Autodesk Fusion 360 part; units mm, degrees
(part 37 of 40)
  line L10333 (174.0805, 208.06) -> (173.9342, 208.1383) construction
  line L10334 (173.9342, 208.1383) -> (173.7873, 208.216) construction
  line L10335 (173.7873, 208.216) -> (173.6399, 208.2931) construction
  line L10336 (173.6399, 208.2931) -> (173.4919, 208.3695) construction
  line L10337 (173.4919, 208.3695) -> (173.3434, 208.4453) construction
  line L10338 (173.3434, 208.4453) -> (173.1943, 208.5205) construction
  line L10339 (173.1943, 208.5205) -> (173.0447, 208.595) construction
  line L10340 (173.0447, 208.595) -> (172.8946, 208.669) construction
  line L10341 (172.8946, 208.669) -> (172.7439, 208.7423) construction
  line L10342 (172.7439, 208.7423) -> (172.5927, 208.8149) construction
  line L10343 (172.5927, 208.8149) -> (172.4411, 208.887) construction
  line L10344 (172.4411, 208.887) -> (172.2889, 208.9584) construction
  line L10345 (172.2889, 208.9584) -> (172.1667, 209.0151) construction
  line L10346 (172.1667, 209.0151) -> (172.0748, 209.0573) construction
  line L10347 (172.0748, 209.0573) -> (172.0135, 209.0853) construction
  line L10348 (172.0135, 209.0853) -> (171.9828, 209.0993) construction
  spline S138 degree 5 poles (217.8271, 89.2315) (217.8299, 89.2007) (217.8349, 89.1391) (217.8398, 89.0467) (217.8417, 88.9234) (217.8376, 88.769) (217.8289, 88.6144) (217.8174, 88.4597) (217.8043, 88.305) (217.7903, 88.1502) (217.7751, 87.9955) (217.7585, 87.8407) (217.74, 87.686) (217.7191, 87.5312) (217.6961, 87.3765) (217.671, 87.2218) (217.6441, 87.0671) (217.6158, 86.9125) (217.5862, 86.7579) (217.5553, 86.6034) (217.5233, 86.4489) (217.4899, 86.2945) (217.4552, 86.1402) (217.4191, 85.986) (217.3817, 85.8318) (217.3429, 85.6778) (217.3029, 85.5238) (217.2617, 85.3699) (217.2193, 85.2161) (217.1759, 85.0624) (217.1313, 84.9088) (217.0856, 84.7553) (217.0388, 84.602) (216.9909, 84.4487) (216.9419, 84.2956) (216.8919, 84.1426) (216.8407, 83.9897) (216.7886, 83.8369) (216.7355, 83.6842) (216.6813, 83.5317) (216.6262, 83.3794) (216.57, 83.2271) (216.513, 83.075) (216.4549, 82.923) (216.3959, 82.7712) (216.3359, 82.6196) (216.275, 82.468) (216.2132, 82.3167) (216.1505, 82.1655) (216.0868, 82.0144) (216.0223, 81.8635) (215.9569, 81.7128) (215.8905, 81.5622) (215.8233, 81.4118) (215.7553, 81.2616) (215.6863, 81.1115) (215.6166, 80.9616) (215.5459, 80.8119) (215.4745, 80.6624) (215.4021, 80.513) (215.329, 80.3638) (215.255, 80.2148) (215.1802, 80.066) (215.1046, 79.9174) (215.0282, 79.7689) (214.951, 79.6207) (214.873, 79.4726) (214.7942, 79.3248) (214.7146, 79.1771) (214.6343, 79.0297) (214.5531, 78.8824) (214.4876, 78.7648) (214.4381, 78.6766) (214.4049, 78.6179) (214.3883, 78.5885) knots 0 0 0 0 0 0 0.01428571 0.02857143 0.04285714 0.05714286 0.07142857 0.08571429 0.1 0.11428571 0.12857143 0.14285714 0.15714286 0.17142857 0.18571429 0.2 0.21428571 0.22857143 0.24285714 0.25714286 0.27142857 0.28571429 0.3 0.31428571 0.32857143 0.34285714 0.35714286 0.37142857 0.38571429 0.4 0.41428571 0.42857143 0.44285714 0.45714286 0.47142857 0.48571429 0.5 0.51428571 0.52857143 0.54285714 0.55714286 0.57142857 0.58571429 0.6 0.61428571 0.62857143 0.64285714 0.65714286 0.67142857 0.68571429 0.7 0.71428571 0.72857143 0.74285714 0.75714286 0.77142857 0.78571429 0.8 0.81428571 0.82857143 0.84285714 0.85714286 0.87142857 0.88571429 0.9 0.91428571 0.92857143 0.94285714 0.95714286 0.97142857 0.98571429 1 1 1 1 1 1
  line L10349 (217.8271, 89.2315) -> (217.8299, 89.2007) construction
  line L10350 (217.8299, 89.2007) -> (217.8349, 89.1391) construction
  line L10351 (217.8349, 89.1391) -> (217.8398, 89.0467) construction
  line L10352 (217.8398, 89.0467) -> (217.8417, 88.9234) construction
  line L10353 (217.8417, 88.9234) -> (217.8376, 88.769) construction
  line L10354 (217.8376, 88.769) -> (217.8289, 88.6144) construction
  line L10355 (217.8289, 88.6144) -> (217.8174, 88.4597) construction
  line L10356 (217.8174, 88.4597) -> (217.8043, 88.305) construction
  line L10357 (217.8043, 88.305) -> (217.7903, 88.1502) construction
  line L10358 (217.7903, 88.1502) -> (217.7751, 87.9955) construction
  line L10359 (217.7751, 87.9955) -> (217.7585, 87.8407) construction
  line L10360 (217.7585, 87.8407) -> (217.74, 87.686) construction
  line L10361 (217.74, 87.686) -> (217.7191, 87.5312) construction
  line L10362 (217.7191, 87.5312) -> (217.6961, 87.3765) construction
  line L10363 (217.6961, 87.3765) -> (217.671, 87.2218) construction
  line L10364 (217.671, 87.2218) -> (217.6441, 87.0671) construction
  line L10365 (217.6441, 87.0671) -> (217.6158, 86.9125) construction
  line L10366 (217.6158, 86.9125) -> (217.5862, 86.7579) construction
  line L10367 (217.5862, 86.7579) -> (217.5553, 86.6034) construction
  line L10368 (217.5553, 86.6034) -> (217.5233, 86.4489) construction
  line L10369 (217.5233, 86.4489) -> (217.4899, 86.2945) construction
  line L10370 (217.4899, 86.2945) -> (217.4552, 86.1402) construction
  line L10371 (217.4552, 86.1402) -> (217.4191, 85.986) construction
  line L10372 (217.4191, 85.986) -> (217.3817, 85.8318) construction
  line L10373 (217.3817, 85.8318) -> (217.3429, 85.6778) construction
  line L10374 (217.3429, 85.6778) -> (217.3029, 85.5238) construction
  line L10375 (217.3029, 85.5238) -> (217.2617, 85.3699) construction
  line L10376 (217.2617, 85.3699) -> (217.2193, 85.2161) construction
  line L10377 (217.2193, 85.2161) -> (217.1759, 85.0624) construction
  line L10378 (217.1759, 85.0624) -> (217.1313, 84.9088) construction
  line L10379 (217.1313, 84.9088) -> (217.0856, 84.7553) construction
  line L10380 (217.0856, 84.7553) -> (217.0388, 84.602) construction
  line L10381 (217.0388, 84.602) -> (216.9909, 84.4487) construction
  line L10382 (216.9909, 84.4487) -> (216.9419, 84.2956) construction
  line L10383 (216.9419, 84.2956) -> (216.8919, 84.1426) construction
  line L10384 (216.8919, 84.1426) -> (216.8407, 83.9897) construction
  line L10385 (216.8407, 83.9897) -> (216.7886, 83.8369) construction
  line L10386 (216.7886, 83.8369) -> (216.7355, 83.6842) construction
  line L10387 (216.7355, 83.6842) -> (216.6813, 83.5317) construction
  line L10388 (216.6813, 83.5317) -> (216.6262, 83.3794) construction
  line L10389 (216.6262, 83.3794) -> (216.57, 83.2271) construction
  line L10390 (216.57, 83.2271) -> (216.513, 83.075) construction
  line L10391 (216.513, 83.075) -> (216.4549, 82.923) construction
  line L10392 (216.4549, 82.923) -> (216.3959, 82.7712) construction
  line L10393 (216.3959, 82.7712) -> (216.3359, 82.6196) construction
  line L10394 (216.3359, 82.6196) -> (216.275, 82.468) construction
  line L10395 (216.275, 82.468) -> (216.2132, 82.3167) construction
  line L10396 (216.2132, 82.3167) -> (216.1505, 82.1655) construction
  line L10397 (216.1505, 82.1655) -> (216.0868, 82.0144) construction
  line L10398 (216.0868, 82.0144) -> (216.0223, 81.8635) construction
  line L10399 (216.0223, 81.8635) -> (215.9569, 81.7128) construction
  line L10400 (215.9569, 81.7128) -> (215.8905, 81.5622) construction
  line L10401 (215.8905, 81.5622) -> (215.8233, 81.4118) construction
  line L10402 (215.8233, 81.4118) -> (215.7553, 81.2616) construction
  line L10403 (215.7553, 81.2616) -> (215.6863, 81.1115) construction
  line L10404 (215.6863, 81.1115) -> (215.6166, 80.9616) construction
  line L10405 (215.6166, 80.9616) -> (215.5459, 80.8119) construction
  line L10406 (215.5459, 80.8119) -> (215.4745, 80.6624) construction
  line L10407 (215.4745, 80.6624) -> (215.4021, 80.513) construction
  line L10408 (215.4021, 80.513) -> (215.329, 80.3638) construction
  line L10409 (215.329, 80.3638) -> (215.255, 80.2148) construction
  line L10410 (215.255, 80.2148) -> (215.1802, 80.066) construction
  line L10411 (215.1802, 80.066) -> (215.1046, 79.9174) construction
  line L10412 (215.1046, 79.9174) -> (215.0282, 79.7689) construction
  line L10413 (215.0282, 79.7689) -> (214.951, 79.6207) construction
  line L10414 (214.951, 79.6207) -> (214.873, 79.4726) construction
  line L10415 (214.873, 79.4726) -> (214.7942, 79.3248) construction
  line L10416 (214.7942, 79.3248) -> (214.7146, 79.1771) construction
  line L10417 (214.7146, 79.1771) -> (214.6343, 79.0297) construction
  line L10418 (214.6343, 79.0297) -> (214.5531, 78.8824) construction
  line L10419 (214.5531, 78.8824) -> (214.4876, 78.7648) construction
  line L10420 (214.4876, 78.7648) -> (214.4381, 78.6766) construction
  line L10421 (214.4381, 78.6766) -> (214.4049, 78.6179) construction
  line L10422 (214.4049, 78.6179) -> (214.3883, 78.5885) construction
  arc A265 (270.0943, 163.005) -> (268.567, 160.6816) centre (270.5321, 161.0535) ccw
  spline S139 degree 5 poles (243.2435, 202.5103) (243.2592, 202.5368) (243.2914, 202.5895) (243.3417, 202.6672) (243.4127, 202.7681) (243.5068, 202.8906) (243.6047, 203.0106) (243.7049, 203.1289) (243.8064, 203.2464) (243.9087, 203.3634) (244.012, 203.4797) (244.1164, 203.5951) (244.2223, 203.7094) (244.3301, 203.8224) (244.4397, 203.934) (244.551, 204.0444) (244.6636, 204.1537) (244.7775, 204.2622) (244.8923, 204.3698) (245.008, 204.4767) (245.1247, 204.5828) (245.2425, 204.6881) (245.3612, 204.7926) (245.4811, 204.8961) (245.602, 204.9988) (245.7239, 205.1007) (245.8468, 205.2017) (245.9706, 205.302) (246.0953, 205.4015) (246.2208, 205.5003) (246.3471, 205.5984) (246.4743, 205.6957) (246.6023, 205.7923) (246.7311, 205.8881) (246.8608, 205.9832) (246.9912, 206.0776) (247.1225, 206.1712) (247.2544, 206.2642) (247.3872, 206.3564) (247.5206, 206.448) (247.6548, 206.5388) (247.7897, 206.629) (247.9253, 206.7185) (248.0615, 206.8073) (248.1985, 206.8955) (248.3362, 206.9829) (248.4745, 207.0697) (248.6135, 207.1558) (248.7531, 207.2413) (248.8934, 207.3261) (249.0343, 207.4102) (249.1758, 207.4937) (249.318, 207.5765) (249.4608, 207.6587) (249.6041, 207.7403) (249.7481, 207.8212) (249.8927, 207.9014) (250.0378, 207.981) (250.1835, 208.06) (250.3298, 208.1383) (250.4767, 208.216) (250.6241, 208.2931) (250.7721, 208.3695) (250.9206, 208.4453) (251.0697, 208.5205) (251.2193, 208.595) (251.3694, 208.669) (251.5201, 208.7423) (251.6713, 208.8149) (251.8229, 208.887) (251.9751, 208.9584) (252.0973, 209.0151) (252.1892, 209.0573) (252.2505, 209.0853) (252.2812, 209.0993) knots 0 0 0 0 0 0 0.01428571 0.02857143 0.04285714 0.05714286 0.07142857 0.08571429 0.1 0.11428571 0.12857143 0.14285714 0.15714286 0.17142857 0.18571429 0.2 0.21428571 0.22857143 0.24285714 0.25714286 0.27142857 0.28571429 0.3 0.31428571 0.32857143 0.34285714 0.35714286 0.37142857 0.38571429 0.4 0.41428571 0.42857143 0.44285714 0.45714286 0.47142857 0.48571429 0.5 0.51428571 0.52857143 0.54285714 0.55714286 0.57142857 0.58571429 0.6 0.61428571 0.62857143 0.64285714 0.65714286 0.67142857 0.68571429 0.7 0.71428571 0.72857143 0.74285714 0.75714286 0.77142857 0.78571429 0.8 0.81428571 0.82857143 0.84285714 0.85714286 0.87142857 0.88571429 0.9 0.91428571 0.92857143 0.94285714 0.95714286 0.97142857 0.98571429 1 1 1 1 1 1
  line L10423 (243.2435, 202.5103) -> (243.2592, 202.5368) construction
  line L10424 (243.2592, 202.5368) -> (243.2914, 202.5895) construction
  line L10425 (243.2914, 202.5895) -> (243.3417, 202.6672) construction
  line L10426 (243.3417, 202.6672) -> (243.4127, 202.7681) construction
  line L10427 (243.4127, 202.7681) -> (243.5068, 202.8906) construction
  line L10428 (243.5068, 202.8906) -> (243.6047, 203.0106) construction
  line L10429 (243.6047, 203.0106) -> (243.7049, 203.1289) construction
  line L10430 (243.7049, 203.1289) -> (243.8064, 203.2464) construction
  line L10431 (243.8064, 203.2464) -> (243.9087, 203.3634) construction
  line L10432 (243.9087, 203.3634) -> (244.012, 203.4797) construction
  line L10433 (244.012, 203.4797) -> (244.1164, 203.5951) construction
  line L10434 (244.1164, 203.5951) -> (244.2223, 203.7094) construction
  line L10435 (244.2223, 203.7094) -> (244.3301, 203.8224) construction
  line L10436 (244.3301, 203.8224) -> (244.4397, 203.934) construction
  line L10437 (244.4397, 203.934) -> (244.551, 204.0444) construction
  line L10438 (244.551, 204.0444) -> (244.6636, 204.1537) construction
  line L10439 (244.6636, 204.1537) -> (244.7775, 204.2622) construction
  line L10440 (244.7775, 204.2622) -> (244.8923, 204.3698) construction
  line L10441 (244.8923, 204.3698) -> (245.008, 204.4767) construction
  line L10442 (245.008, 204.4767) -> (245.1247, 204.5828) construction
  line L10443 (245.1247, 204.5828) -> (245.2425, 204.6881) construction
  line L10444 (245.2425, 204.6881) -> (245.3612, 204.7926) construction
  line L10445 (245.3612, 204.7926) -> (245.4811, 204.8961) construction
  line L10446 (245.4811, 204.8961) -> (245.602, 204.9988) construction
  line L10447 (245.602, 204.9988) -> (245.7239, 205.1007) construction
  line L10448 (245.7239, 205.1007) -> (245.8468, 205.2017) construction
  line L10449 (245.8468, 205.2017) -> (245.9706, 205.302) construction
  line L10450 (245.9706, 205.302) -> (246.0953, 205.4015) construction
  line L10451 (246.0953, 205.4015) -> (246.2208, 205.5003) construction
  line L10452 (246.2208, 205.5003) -> (246.3471, 205.5984) construction
  line L10453 (246.3471, 205.5984) -> (246.4743, 205.6957) construction
  line L10454 (246.4743, 205.6957) -> (246.6023, 205.7923) construction
  line L10455 (246.6023, 205.7923) -> (246.7311, 205.8881) construction
  line L10456 (246.7311, 205.8881) -> (246.8608, 205.9832) construction
  line L10457 (246.8608, 205.9832) -> (246.9912, 206.0776) construction
  line L10458 (246.9912, 206.0776) -> (247.1225, 206.1712) construction
  line L10459 (247.1225, 206.1712) -> (247.2544, 206.2642) construction
  line L10460 (247.2544, 206.2642) -> (247.3872, 206.3564) construction
  line L10461 (247.3872, 206.3564) -> (247.5206, 206.448) construction
  line L10462 (247.5206, 206.448) -> (247.6548, 206.5388) construction
  line L10463 (247.6548, 206.5388) -> (247.7897, 206.629) construction
  line L10464 (247.7897, 206.629) -> (247.9253, 206.7185) construction
  line L10465 (247.9253, 206.7185) -> (248.0615, 206.8073) construction
  line L10466 (248.0615, 206.8073) -> (248.1985, 206.8955) construction
  line L10467 (248.1985, 206.8955) -> (248.3362, 206.9829) construction
  line L10468 (248.3362, 206.9829) -> (248.4745, 207.0697) construction
  line L10469 (248.4745, 207.0697) -> (248.6135, 207.1558) construction
  line L10470 (248.6135, 207.1558) -> (248.7531, 207.2413) construction
  line L10471 (248.7531, 207.2413) -> (248.8934, 207.3261) construction
  line L10472 (248.8934, 207.3261) -> (249.0343, 207.4102) construction
  line L10473 (249.0343, 207.4102) -> (249.1758, 207.4937) construction
  line L10474 (249.1758, 207.4937) -> (249.318, 207.5765) construction
  line L10475 (249.318, 207.5765) -> (249.4608, 207.6587) construction
  line L10476 (249.4608, 207.6587) -> (249.6041, 207.7403) construction
  line L10477 (249.6041, 207.7403) -> (249.7481, 207.8212) construction
  line L10478 (249.7481, 207.8212) -> (249.8927, 207.9014) construction
  line L10479 (249.8927, 207.9014) -> (250.0378, 207.981) construction
  line L10480 (250.0378, 207.981) -> (250.1835, 208.06) construction
  line L10481 (250.1835, 208.06) -> (250.3298, 208.1383) construction
  line L10482 (250.3298, 208.1383) -> (250.4767, 208.216) construction
  line L10483 (250.4767, 208.216) -> (250.6241, 208.2931) construction
  line L10484 (250.6241, 208.2931) -> (250.7721, 208.3695) construction
  line L10485 (250.7721, 208.3695) -> (250.9206, 208.4453) construction
  line L10486 (250.9206, 208.4453) -> (251.0697, 208.5205) construction
  line L10487 (251.0697, 208.5205) -> (251.2193, 208.595) construction
  line L10488 (251.2193, 208.595) -> (251.3694, 208.669) construction
  line L10489 (251.3694, 208.669) -> (251.5201, 208.7423) construction
  line L10490 (251.5201, 208.7423) -> (251.6713, 208.8149) construction
  line L10491 (251.6713, 208.8149) -> (251.8229, 208.887) construction
  line L10492 (251.8229, 208.887) -> (251.9751, 208.9584) construction
  line L10493 (251.9751, 208.9584) -> (252.0973, 209.0151) construction
  line L10494 (252.0973, 209.0151) -> (252.1892, 209.0573) construction
  line L10495 (252.1892, 209.0573) -> (252.2505, 209.0853) construction
  line L10496 (252.2505, 209.0853) -> (252.2812, 209.0993) construction
  arc A266 (217.6748, 209.1442) -> (219.4126, 206.9737) centre (219.6661, 208.9575) ccw
  arc A267 (140.7205, 152.2563) -> (140.7205, 147.7437) centre (212.132, 150) ccw
  line L10497 (152.9878, 144.4572) -> (151.3635, 144.3049)
  arc A268 (160.1966, 125.4699) -> (157.5954, 126.4519) centre (158.3882, 124.6158) ccw
  line L10498 (263.2386, 119.7202) -> (264.6423, 118.8885)
  line L10499 (242.4118, 98.8934) -> (243.2435, 97.4897)
  line L10500 (154.1697, 163.005) -> (152.5778, 163.3622)
  arc A269 (256.7226, 110.7517) -> (253.9452, 110.6216) centre (255.4012, 109.2504) ccw
  arc A270 (168.332, 93.5531) -> (171.9828, 90.9007) centre (212.132, 150) ccw
  arc A271 (271.2313, 190.1492) -> (268.5789, 193.8) centre (212.132, 150) ccw
  arc A272 (187.6019, 201.9354) -> (184.5338, 200.3721) centre (212.132, 150) ccw
  arc A273 (188.5839, 95.4634) -> (187.6019, 98.0646) centre (186.7478, 96.2562) ccw
  arc A274 (161.7599, 177.5982) -> (161.0254, 180.2798) centre (160.0059, 178.5592) ccw
  arc A275 (253.9452, 189.3784) -> (256.7226, 189.2483) centre (255.4012, 190.7496) ccw
  arc A276 (153.0327, 109.8508) -> (155.6851, 106.2) centre (212.132, 150) ccw
  arc A277 (184.5338, 99.6279) -> (181.8522, 98.8934) centre (183.5728, 97.8739) ccw
  arc A278 (263.2386, 180.2798) -> (262.5041, 177.5982) centre (264.2581, 178.5592) ccw
  arc A279 (264.0674, 174.5301) -> (262.5041, 177.5982) centre (212.132, 150) ccw
  spline S140 degree 5 poles (152.5778, 163.3622) (152.5477, 163.369) (152.4876, 163.3833) (152.3982, 163.4071) (152.2803, 163.4435) (152.1347, 163.4951) (151.9904, 163.5511) (151.8468, 163.6099) (151.7037, 163.6701) (151.5609, 163.7313) (151.4184, 163.7935) (151.2763, 163.8571) (151.1349, 163.9226) (150.9941, 163.9902) (150.8541, 164.06) (150.7147, 164.1316) (150.5759, 164.205) (150.4376, 164.2797) (150.2998, 164.3557) (150.1623, 164.4327) (150.0253, 164.5109) (149.8888, 164.5904) (149.7528, 164.6711) (149.6172, 164.753) (149.4822, 164.8363) (149.3477, 164.9208) (149.2136, 165.0064) (149.08, 165.0932) (148.9468, 165.181) (148.814, 165.2698) (148.6817, 165.3597) (148.5499, 165.4506) (148.4185, 165.5425) (148.2875, 165.6354) (148.157, 165.7293) (148.027, 165.8242) (147.8974, 165.92) (147.7682, 166.0168) (147.6394, 166.1146) (147.5111, 166.2132) (147.3832, 166.3127) (147.2558, 166.4131) (147.1288, 166.5144) (147.0022, 166.6166) (146.876, 166.7196) (146.7503, 166.8235) (146.625, 166.9283) (146.5002, 167.0338) (146.3758, 167.1402) (146.2518, 167.2474) (146.1282, 167.3555) (146.0051, 167.4643) (145.8823, 167.5739) (145.7601, 167.6842) (145.6382, 167.7954) (145.5168, 167.9073) (145.3958, 168.02) (145.2752, 168.1335) (145.1551, 168.2477) (145.0354, 168.3626) (144.9161, 168.4782) (144.7973, 168.5946) (144.6789, 168.7118) (144.5609, 168.8296) (144.4433, 168.9481) (144.3262, 169.0674) (144.2095, 169.1873) (144.0932, 169.3079) (143.9774, 169.4293) (143.862, 169.5512) (143.747, 169.6739) (143.6553, 169.7726) (143.5868, 169.8469) (143.5412, 169.8966) (143.5184, 169.9215) knots 0 0 0 0 0 0 0.01428571 0.02857143 0.04285714 0.05714286 0.07142857 0.08571429 0.1 0.11428571 0.12857143 0.14285714 0.15714286 0.17142857 0.18571429 0.2 0.21428571 0.22857143 0.24285714 0.25714286 0.27142857 0.28571429 0.3 0.31428571 0.32857143 0.34285714 0.35714286 0.37142857 0.38571429 0.4 0.41428571 0.42857143 0.44285714 0.45714286 0.47142857 0.48571429 0.5 0.51428571 0.52857143 0.54285714 0.55714286 0.57142857 0.58571429 0.6 0.61428571 0.62857143 0.64285714 0.65714286 0.67142857 0.68571429 0.7 0.71428571 0.72857143 0.74285714 0.75714286 0.77142857 0.78571429 0.8 0.81428571 0.82857143 0.84285714 0.85714286 0.87142857 0.88571429 0.9 0.91428571 0.92857143 0.94285714 0.95714286 0.97142857 0.98571429 1 1 1 1 1 1
  line L10501 (152.5778, 163.3622) -> (152.5477, 163.369) construction
  line L10502 (152.5477, 163.369) -> (152.4876, 163.3833) construction
  line L10503 (152.4876, 163.3833) -> (152.3982, 163.4071) construction
  line L10504 (152.3982, 163.4071) -> (152.2803, 163.4435) construction
  line L10505 (152.2803, 163.4435) -> (152.1347, 163.4951) construction
  line L10506 (152.1347, 163.4951) -> (151.9904, 163.5511) construction
  line L10507 (151.9904, 163.5511) -> (151.8468, 163.6099) construction
  line L10508 (151.8468, 163.6099) -> (151.7037, 163.6701) construction
  line L10509 (151.7037, 163.6701) -> (151.5609, 163.7313) construction
  line L10510 (151.5609, 163.7313) -> (151.4184, 163.7935) construction
  line L10511 (151.4184, 163.7935) -> (151.2763, 163.8571) construction
  line L10512 (151.2763, 163.8571) -> (151.1349, 163.9226) construction
  line L10513 (151.1349, 163.9226) -> (150.9941, 163.9902) construction
  line L10514 (150.9941, 163.9902) -> (150.8541, 164.06) construction
  line L10515 (150.8541, 164.06) -> (150.7147, 164.1316) construction
  line L10516 (150.7147, 164.1316) -> (150.5759, 164.205) construction
  line L10517 (150.5759, 164.205) -> (150.4376, 164.2797) construction
  line L10518 (150.4376, 164.2797) -> (150.2998, 164.3557) construction
  line L10519 (150.2998, 164.3557) -> (150.1623, 164.4327) construction
  line L10520 (150.1623, 164.4327) -> (150.0253, 164.5109) construction
  line L10521 (150.0253, 164.5109) -> (149.8888, 164.5904) construction
  line L10522 (149.8888, 164.5904) -> (149.7528, 164.6711) construction
  line L10523 (149.7528, 164.6711) -> (149.6172, 164.753) construction
  line L10524 (149.6172, 164.753) -> (149.4822, 164.8363) construction
  line L10525 (149.4822, 164.8363) -> (149.3477, 164.9208) construction
  line L10526 (149.3477, 164.9208) -> (149.2136, 165.0064) construction
  line L10527 (149.2136, 165.0064) -> (149.08, 165.0932) construction
  line L10528 (149.08, 165.0932) -> (148.9468, 165.181) construction
  line L10529 (148.9468, 165.181) -> (148.814, 165.2698) construction
  line L10530 (148.814, 165.2698) -> (148.6817, 165.3597) construction
  line L10531 (148.6817, 165.3597) -> (148.5499, 165.4506) construction
  line L10532 (148.5499, 165.4506) -> (148.4185, 165.5425) construction
  line L10533 (148.4185, 165.5425) -> (148.2875, 165.6354) construction
  line L10534 (148.2875, 165.6354) -> (148.157, 165.7293) construction
  line L10535 (148.157, 165.7293) -> (148.027, 165.8242) construction
  line L10536 (148.027, 165.8242) -> (147.8974, 165.92) construction
  line L10537 (147.8974, 165.92) -> (147.7682, 166.0168) construction
  line L10538 (147.7682, 166.0168) -> (147.6394, 166.1146) construction
  line L10539 (147.6394, 166.1146) -> (147.5111, 166.2132) construction
  line L10540 (147.5111, 166.2132) -> (147.3832, 166.3127) construction
  line L10541 (147.3832, 166.3127) -> (147.2558, 166.4131) construction
  line L10542 (147.2558, 166.4131) -> (147.1288, 166.5144) construction
  line L10543 (147.1288, 166.5144) -> (147.0022, 166.6166) construction
  line L10544 (147.0022, 166.6166) -> (146.876, 166.7196) construction
  line L10545 (146.876, 166.7196) -> (146.7503, 166.8235) construction
  line L10546 (146.7503, 166.8235) -> (146.625, 166.9283) construction
  line L10547 (146.625, 166.9283) -> (146.5002, 167.0338) construction
  line L10548 (146.5002, 167.0338) -> (146.3758, 167.1402) construction
  line L10549 (146.3758, 167.1402) -> (146.2518, 167.2474) construction
  line L10550 (146.2518, 167.2474) -> (146.1282, 167.3555) construction
  line L10551 (146.1282, 167.3555) -> (146.0051, 167.4643) construction
  line L10552 (146.0051, 167.4643) -> (145.8823, 167.5739) construction
  line L10553 (145.8823, 167.5739) -> (145.7601, 167.6842) construction
  line L10554 (145.7601, 167.6842) -> (145.6382, 167.7954) construction
  line L10555 (145.6382, 167.7954) -> (145.5168, 167.9073) construction
  line L10556 (145.5168, 167.9073) -> (145.3958, 168.02) construction
  line L10557 (145.3958, 168.02) -> (145.2752, 168.1335) construction
  line L10558 (145.2752, 168.1335) -> (145.1551, 168.2477) construction
  line L10559 (145.1551, 168.2477) -> (145.0354, 168.3626) construction
  line L10560 (145.0354, 168.3626) -> (144.9161, 168.4782) construction
  line L10561 (144.9161, 168.4782) -> (144.7973, 168.5946) construction
  line L10562 (144.7973, 168.5946) -> (144.6789, 168.7118) construction
  line L10563 (144.6789, 168.7118) -> (144.5609, 168.8296) construction
  line L10564 (144.5609, 168.8296) -> (144.4433, 168.9481) construction
  line L10565 (144.4433, 168.9481) -> (144.3262, 169.0674) construction
  line L10566 (144.3262, 169.0674) -> (144.2095, 169.1873) construction
  line L10567 (144.2095, 169.1873) -> (144.0932, 169.3079) construction
  line L10568 (144.0932, 169.3079) -> (143.9774, 169.4293) construction
  line L10569 (143.9774, 169.4293) -> (143.862, 169.5512) construction
  line L10570 (143.862, 169.5512) -> (143.747, 169.6739) construction
  line L10571 (143.747, 169.6739) -> (143.6553, 169.7726) construction
  line L10572 (143.6553, 169.7726) -> (143.5868, 169.8469) construction
  line L10573 (143.5868, 169.8469) -> (143.5412, 169.8966) construction
  line L10574 (143.5412, 169.8966) -> (143.5184, 169.9215) construction
  arc A280 (184.5338, 99.6279) -> (187.6019, 98.0646) centre (212.132, 150) ccw
  arc A281 (268.567, 139.3184) -> (269.1057, 142.7194) centre (212.132, 150) ccw
  arc A282 (160.1966, 125.4699) -> (161.7599, 122.4018) centre (212.132, 150) ccw
  spline S141 degree 5 poles (243.2435, 202.5103) (243.2592, 202.5368) (243.2914, 202.5895) (243.3417, 202.6672) (243.4127, 202.7681) (243.5068, 202.8906) (243.6047, 203.0106) (243.7049, 203.1289) (243.8064, 203.2464) (243.9087, 203.3634) (244.012, 203.4797) (244.1164, 203.5951) (244.2223, 203.7094) (244.3301, 203.8224) (244.4397, 203.934) (244.551, 204.0444) (244.6636, 204.1537) (244.7775, 204.2622) (244.8923, 204.3698) (245.008, 204.4767) (245.1247, 204.5828) (245.2425, 204.6881) (245.3612, 204.7926) (245.4811, 204.8961) (245.602, 204.9988) (245.7239, 205.1007) (245.8468, 205.2017) (245.9706, 205.302) (246.0953, 205.4015) (246.2208, 205.5003) (246.3471, 205.5984) (246.4743, 205.6957) (246.6023, 205.7923) (246.7311, 205.8881) (246.8608, 205.9832) (246.9912, 206.0776) (247.1225, 206.1712) (247.2544, 206.2642) (247.3872, 206.3564) (247.5206, 206.448) (247.6548, 206.5388) (247.7897, 206.629) (247.9253, 206.7185) (248.0615, 206.8073) (248.1985, 206.8955) (248.3362, 206.9829) (248.4745, 207.0697) (248.6135, 207.1558) (248.7531, 207.2413) (248.8934, 207.3261) (249.0343, 207.4102) (249.1758, 207.4937) (249.318, 207.5765) (249.4608, 207.6587) (249.6041, 207.7403) (249.7481, 207.8212) (249.8927, 207.9014) (250.0378, 207.981) (250.1835, 208.06) (250.3298, 208.1383) (250.4767, 208.216) (250.6241, 208.2931) (250.7721, 208.3695) (250.9206, 208.4453) (251.0697, 208.5205) (251.2193, 208.595) (251.3694, 208.669) (251.5201, 208.7423) (251.6713, 208.8149) (251.8229, 208.887) (251.9751, 208.9584) (252.0973, 209.0151) (252.1892, 209.0573) (252.2505, 209.0853) (252.2812, 209.0993) knots 0 0 0 0 0 0 0.01428571 0.02857143 0.04285714 0.05714286 0.07142857 0.08571429 0.1 0.11428571 0.12857143 0.14285714 0.15714286 0.17142857 0.18571429 0.2 0.21428571 0.22857143 0.24285714 0.25714286 0.27142857 0.28571429 0.3 0.31428571 0.32857143 0.34285714 0.35714286 0.37142857 0.38571429 0.4 0.41428571 0.42857143 0.44285714 0.45714286 0.47142857 0.48571429 0.5 0.51428571 0.52857143 0.54285714 0.55714286 0.57142857 0.58571429 0.6 0.61428571 0.62857143 0.64285714 0.65714286 0.67142857 0.68571429 0.7 0.71428571 0.72857143 0.74285714 0.75714286 0.77142857 0.78571429 0.8 0.81428571 0.82857143 0.84285714 0.85714286 0.87142857 0.88571429 0.9 0.91428571 0.92857143 0.94285714 0.95714286 0.97142857 0.98571429 1 1 1 1 1 1
  line L10575 (243.2435, 202.5103) -> (243.2592, 202.5368) construction
  line L10576 (243.2592, 202.5368) -> (243.2914, 202.5895) construction
  line L10577 (243.2914, 202.5895) -> (243.3417, 202.6672) construction
  line L10578 (243.3417, 202.6672) -> (243.4127, 202.7681) construction
  line L10579 (243.4127, 202.7681) -> (243.5068, 202.8906) construction
  line L10580 (243.5068, 202.8906) -> (243.6047, 203.0106) construction
  line L10581 (243.6047, 203.0106) -> (243.7049, 203.1289) construction
  line L10582 (243.7049, 203.1289) -> (243.8064, 203.2464) construction
  line L10583 (243.8064, 203.2464) -> (243.9087, 203.3634) construction
  line L10584 (243.9087, 203.3634) -> (244.012, 203.4797) construction
  line L10585 (244.012, 203.4797) -> (244.1164, 203.5951) construction
  line L10586 (244.1164, 203.5951) -> (244.2223, 203.7094) construction
  line L10587 (244.2223, 203.7094) -> (244.3301, 203.8224) construction
  line L10588 (244.3301, 203.8224) -> (244.4397, 203.934) construction
  line L10589 (244.4397, 203.934) -> (244.551, 204.0444) construction
  line L10590 (244.551, 204.0444) -> (244.6636, 204.1537) construction
  line L10591 (244.6636, 204.1537) -> (244.7775, 204.2622) construction
  line L10592 (244.7775, 204.2622) -> (244.8923, 204.3698) construction
  line L10593 (244.8923, 204.3698) -> (245.008, 204.4767) construction
  line L10594 (245.008, 204.4767) -> (245.1247, 204.5828) construction
  line L10595 (245.1247, 204.5828) -> (245.2425, 204.6881) construction
  line L10596 (245.2425, 204.6881) -> (245.3612, 204.7926) construction
  line L10597 (245.3612, 204.7926) -> (245.4811, 204.8961) construction
  line L10598 (245.4811, 204.8961) -> (245.602, 204.9988) construction
  line L10599 (245.602, 204.9988) -> (245.7239, 205.1007) construction
  line L10600 (245.7239, 205.1007) -> (245.8468, 205.2017) construction
  line L10601 (245.8468, 205.2017) -> (245.9706, 205.302) construction
  line L10602 (245.9706, 205.302) -> (246.0953, 205.4015) construction
  line L10603 (246.0953, 205.4015) -> (246.2208, 205.5003) construction
  line L10604 (246.2208, 205.5003) -> (246.3471, 205.5984) construction
  line L10605 (246.3471, 205.5984) -> (246.4743, 205.6957) construction
  line L10606 (246.4743, 205.6957) -> (246.6023, 205.7923) construction
  line L10607 (246.6023, 205.7923) -> (246.7311, 205.8881) construction
  line L10608 (246.7311, 205.8881) -> (246.8608, 205.9832) construction
  line L10609 (246.8608, 205.9832) -> (246.9912, 206.0776) construction
  line L10610 (246.9912, 206.0776) -> (247.1225, 206.1712) construction
  line L10611 (247.1225, 206.1712) -> (247.2544, 206.2642) construction
  line L10612 (247.2544, 206.2642) -> (247.3872, 206.3564) construction
  line L10613 (247.3872, 206.3564) -> (247.5206, 206.448) construction
  line L10614 (247.5206, 206.448) -> (247.6548, 206.5388) construction
  line L10615 (247.6548, 206.5388) -> (247.7897, 206.629) construction
  line L10616 (247.7897, 206.629) -> (247.9253, 206.7185) construction
  line L10617 (247.9253, 206.7185) -> (248.0615, 206.8073) construction
  line L10618 (248.0615, 206.8073) -> (248.1985, 206.8955) construction
  line L10619 (248.1985, 206.8955) -> (248.3362, 206.9829) construction
  line L10620 (248.3362, 206.9829) -> (248.4745, 207.0697) construction
  line L10621 (248.4745, 207.0697) -> (248.6135, 207.1558) construction
  line L10622 (248.6135, 207.1558) -> (248.7531, 207.2413) construction
  line L10623 (248.7531, 207.2413) -> (248.8934, 207.3261) construction
  line L10624 (248.8934, 207.3261) -> (249.0343, 207.4102) construction
  line L10625 (249.0343, 207.4102) -> (249.1758, 207.4937) construction
  line L10626 (249.1758, 207.4937) -> (249.318, 207.5765) construction
  line L10627 (249.318, 207.5765) -> (249.4608, 207.6587) construction
  line L10628 (249.4608, 207.6587) -> (249.6041, 207.7403) construction
  line L10629 (249.6041, 207.7403) -> (249.7481, 207.8212) construction
  line L10630 (249.7481, 207.8212) -> (249.8927, 207.9014) construction
  line L10631 (249.8927, 207.9014) -> (250.0378, 207.981) construction
  line L10632 (250.0378, 207.981) -> (250.1835, 208.06) construction
  line L10633 (250.1835, 208.06) -> (250.3298, 208.1383) construction
  line L10634 (250.3298, 208.1383) -> (250.4767, 208.216) construction
  line L10635 (250.4767, 208.216) -> (250.6241, 208.2931) construction
  line L10636 (250.6241, 208.2931) -> (250.7721, 208.3695) construction
  line L10637 (250.7721, 208.3695) -> (250.9206, 208.4453) construction
  line L10638 (250.9206, 208.4453) -> (251.0697, 208.5205) construction
  line L10639 (251.0697, 208.5205) -> (251.2193, 208.595) construction
  line L10640 (251.2193, 208.595) -> (251.3694, 208.669) construction
  line L10641 (251.3694, 208.669) -> (251.5201, 208.7423) construction
  line L10642 (251.5201, 208.7423) -> (251.6713, 208.8149) construction
  line L10643 (251.6713, 208.8149) -> (251.8229, 208.887) construction
  line L10644 (251.8229, 208.887) -> (251.9751, 208.9584) construction
  line L10645 (251.9751, 208.9584) -> (252.0973, 209.0151) construction
  line L10646 (252.0973, 209.0151) -> (252.1892, 209.0573) construction
  line L10647 (252.1892, 209.0573) -> (252.2505, 209.0853) construction
  line L10648 (252.2505, 209.0853) -> (252.2812, 209.0993) construction
  spline S142 degree 5 poles (187.9372, 206.0345) (187.9249, 206.0628) (187.9012, 206.1198) (187.868, 206.2062) (187.8281, 206.3229) (187.7842, 206.4711) (187.7447, 206.6208) (187.7079, 206.7714) (187.6725, 206.9226) (187.638, 207.0741) (187.6046, 207.226) (187.5726, 207.3783) (187.5424, 207.5312) (187.5144, 207.6848) (187.4885, 207.8391) (187.4646, 207.994) (187.4423, 208.1494) (187.4215, 208.3052) (187.4019, 208.4614) (187.3835, 208.6179) (187.3662, 208.7747) (187.3502, 208.9318) (187.3355, 209.0893) (187.3222, 209.2471) (187.3102, 209.4053) (187.2995, 209.5638) (187.29, 209.7226) (187.2816, 209.8817) (187.2743, 210.0411) (187.2682, 210.2007) (187.2631, 210.3605) (187.2591, 210.5206) (187.2563, 210.6809) (187.2544, 210.8415) (187.2537, 211.0023) (187.254, 211.1633) (187.2554, 211.3245) (187.2578, 211.4859) (187.2612, 211.6475) (187.2655, 211.8093) (187.2709, 211.9712) (187.2772, 212.1334) (187.2845, 212.2957) (187.2928, 212.4581) (187.302, 212.6207) (187.3121, 212.7835) (187.3232, 212.9464) (187.3353, 213.1095) (187.3482, 213.2727) (187.362, 213.436) (187.3768, 213.5995) (187.3924, 213.7631) (187.409, 213.9268) (187.4264, 214.0906) (187.4447, 214.2545) (187.4639, 214.4185) (187.484, 214.5826) (187.5049, 214.7468) (187.5266, 214.9111) (187.5492, 215.0755) (187.5727, 215.24) (187.597, 215.4046) (187.6222, 215.5692) (187.6481, 215.734) (187.6749, 215.8987) (187.7026, 216.0636) (187.731, 216.2285) (187.7602, 216.3935) (187.7903, 216.5585) (187.8212, 216.7236) (187.8528, 216.8887) (187.8788, 217.0208) (187.8986, 217.1199) (187.912, 217.186) (187.9188, 217.2191) knots 0 0 0 0 0 0 0.01428571 0.02857143 0.04285714 0.05714286 0.07142857 0.08571429 0.1 0.11428571 0.12857143 0.14285714 0.15714286 0.17142857 0.18571429 0.2 0.21428571 0.22857143 0.24285714 0.25714286 0.27142857 0.28571429 0.3 0.31428571 0.32857143 0.34285714 0.35714286 0.37142857 0.38571429 0.4 0.41428571 0.42857143 0.44285714 0.45714286 0.47142857 0.48571429 0.5 0.51428571 0.52857143 0.54285714 0.55714286 0.57142857 0.58571429 0.6 0.61428571 0.62857143 0.64285714 0.65714286 0.67142857 0.68571429 0.7 0.71428571 0.72857143 0.74285714 0.75714286 0.77142857 0.78571429 0.8 0.81428571 0.82857143 0.84285714 0.85714286 0.87142857 0.88571429 0.9 0.91428571 0.92857143 0.94285714 0.95714286 0.97142857 0.98571429 1 1 1 1 1 1
  line L10649 (187.9372, 206.0345) -> (187.9249, 206.0628) construction
  line L10650 (187.9249, 206.0628) -> (187.9012, 206.1198) construction
  line L10651 (187.9012, 206.1198) -> (187.868, 206.2062) construction
  line L10652 (187.868, 206.2062) -> (187.8281, 206.3229) construction
  line L10653 (187.8281, 206.3229) -> (187.7842, 206.4711) construction
  line L10654 (187.7842, 206.4711) -> (187.7447, 206.6208) construction
  line L10655 (187.7447, 206.6208) -> (187.7079, 206.7714) construction
  line L10656 (187.7079, 206.7714) -> (187.6725, 206.9226) construction
  line L10657 (187.6725, 206.9226) -> (187.638, 207.0741) construction
  line L10658 (187.638, 207.0741) -> (187.6046, 207.226) construction
  line L10659 (187.6046, 207.226) -> (187.5726, 207.3783) construction
  line L10660 (187.5726, 207.3783) -> (187.5424, 207.5312) construction
  line L10661 (187.5424, 207.5312) -> (187.5144, 207.6848) construction
  line L10662 (187.5144, 207.6848) -> (187.4885, 207.8391) construction
  line L10663 (187.4885, 207.8391) -> (187.4646, 207.994) construction
  line L10664 (187.4646, 207.994) -> (187.4423, 208.1494) construction
  line L10665 (187.4423, 208.1494) -> (187.4215, 208.3052) construction
  line L10666 (187.4215, 208.3052) -> (187.4019, 208.4614) construction
  line L10667 (187.4019, 208.4614) -> (187.3835, 208.6179) construction
  line L10668 (187.3835, 208.6179) -> (187.3662, 208.7747) construction
  line L10669 (187.3662, 208.7747) -> (187.3502, 208.9318) construction
  line L10670 (187.3502, 208.9318) -> (187.3355, 209.0893) construction
  line L10671 (187.3355, 209.0893) -> (187.3222, 209.2471) construction
  line L10672 (187.3222, 209.2471) -> (187.3102, 209.4053) construction
  line L10673 (187.3102, 209.4053) -> (187.2995, 209.5638) construction
  line L10674 (187.2995, 209.5638) -> (187.29, 209.7226) construction
  line L10675 (187.29, 209.7226) -> (187.2816, 209.8817) construction
  line L10676 (187.2816, 209.8817) -> (187.2743, 210.0411) construction
  line L10677 (187.2743, 210.0411) -> (187.2682, 210.2007) construction
  line L10678 (187.2682, 210.2007) -> (187.2631, 210.3605) construction
  line L10679 (187.2631, 210.3605) -> (187.2591, 210.5206) construction
  line L10680 (187.2591, 210.5206) -> (187.2563, 210.6809) construction
  line L10681 (187.2563, 210.6809) -> (187.2544, 210.8415) construction
  line L10682 (187.2544, 210.8415) -> (187.2537, 211.0023) construction
  line L10683 (187.2537, 211.0023) -> (187.254, 211.1633) construction
  line L10684 (187.254, 211.1633) -> (187.2554, 211.3245) construction
  line L10685 (187.2554, 211.3245) -> (187.2578, 211.4859) construction
  line L10686 (187.2578, 211.4859) -> (187.2612, 211.6475) construction
  line L10687 (187.2612, 211.6475) -> (187.2655, 211.8093) construction
  line L10688 (187.2655, 211.8093) -> (187.2709, 211.9712) construction
  line L10689 (187.2709, 211.9712) -> (187.2772, 212.1334) construction
  line L10690 (187.2772, 212.1334) -> (187.2845, 212.2957) construction
  line L10691 (187.2845, 212.2957) -> (187.2928, 212.4581) construction
  line L10692 (187.2928, 212.4581) -> (187.302, 212.6207) construction
  line L10693 (187.302, 212.6207) -> (187.3121, 212.7835) construction
  line L10694 (187.3121, 212.7835) -> (187.3232, 212.9464) construction
  line L10695 (187.3232, 212.9464) -> (187.3353, 213.1095) construction
  line L10696 (187.3353, 213.1095) -> (187.3482, 213.2727) construction
  line L10697 (187.3482, 213.2727) -> (187.362, 213.436) construction
  line L10698 (187.362, 213.436) -> (187.3768, 213.5995) construction
  line L10699 (187.3768, 213.5995) -> (187.3924, 213.7631) construction
  line L10700 (187.3924, 213.7631) -> (187.409, 213.9268) construction
  line L10701 (187.409, 213.9268) -> (187.4264, 214.0906) construction
  line L10702 (187.4264, 214.0906) -> (187.4447, 214.2545) construction
  line L10703 (187.4447, 214.2545) -> (187.4639, 214.4185) construction
  line L10704 (187.4639, 214.4185) -> (187.484, 214.5826) construction
  line L10705 (187.484, 214.5826) -> (187.5049, 214.7468) construction
  line L10706 (187.5049, 214.7468) -> (187.5266, 214.9111) construction
  line L10707 (187.5266, 214.9111) -> (187.5492, 215.0755) construction
  line L10708 (187.5492, 215.0755) -> (187.5727, 215.24) construction
  line L10709 (187.5727, 215.24) -> (187.597, 215.4046) construction
  line L10710 (187.597, 215.4046) -> (187.6222, 215.5692) construction
  line L10711 (187.6222, 215.5692) -> (187.6481, 215.734) construction
  line L10712 (187.6481, 215.734) -> (187.6749, 215.8987) construction
  line L10713 (187.6749, 215.8987) -> (187.7026, 216.0636) construction
  line L10714 (187.7026, 216.0636) -> (187.731, 216.2285) construction
  line L10715 (187.731, 216.2285) -> (187.7602, 216.3935) construction
  line L10716 (187.7602, 216.3935) -> (187.7903, 216.5585) construction
  line L10717 (187.7903, 216.5585) -> (187.8212, 216.7236) construction
  line L10718 (187.8212, 216.7236) -> (187.8528, 216.8887) construction
  line L10719 (187.8528, 216.8887) -> (187.8788, 217.0208) construction
  line L10720 (187.8788, 217.0208) -> (187.8986, 217.1199) construction
  line L10721 (187.8986, 217.1199) -> (187.912, 217.186) construction
  line L10722 (187.912, 217.186) -> (187.9188, 217.2191) construction
  spline S143 degree 5 poles (166.3167, 190.3263) (166.2935, 190.3467) (166.2466, 190.3868) (166.1747, 190.4451) (166.076, 190.5192) (165.9487, 190.6066) (165.8185, 190.6904) (165.6866, 190.772) (165.5538, 190.8524) (165.4203, 190.932) (165.2862, 191.0107) (165.1513, 191.0883) (165.0152, 191.1642) (164.8777, 191.2383) (164.739, 191.3106) (164.5991, 191.3813) (164.4582, 191.4504) (164.3164, 191.5184) (164.1739, 191.5853) (164.0308, 191.6512) (163.887, 191.716) (163.7425, 191.7798) (163.5973, 191.8424) (163.4513, 191.9039) (163.3046, 191.9642) (163.1571, 192.0234) (163.009, 192.0815) (162.8603, 192.1386) (162.711, 192.1947) (162.5611, 192.2499) (162.4106, 192.3041) (162.2596, 192.3574) (162.108, 192.4097) (161.9559, 192.461) (161.8032, 192.5114) (161.65, 192.5608) (161.4962, 192.6094) (161.342, 192.657) (161.1873, 192.7037) (161.0321, 192.7495) (160.8764, 192.7945) (160.7202, 192.8386) (160.5636, 192.8818) (160.4065, 192.9241) (160.249, 192.9656) (160.0911, 193.0063) (159.9327, 193.0461) (159.7739, 193.085) (159.6147, 193.1231) (159.4551, 193.1604) (159.2951, 193.1969) (159.1347, 193.2326) (158.9739, 193.2674) (158.8127, 193.3015) (158.6511, 193.3347) (158.4892, 193.3672) (158.3269, 193.3988) (158.1643, 193.4297) (158.0013, 193.4597) (157.838, 193.489) (157.6743, 193.5175) (157.5103, 193.5453) (157.3459, 193.5723) (157.1812, 193.5984) (157.0162, 193.6239) (156.8509, 193.6486) (156.6853, 193.6725) (156.5194, 193.6956) (156.3531, 193.718) (156.1866, 193.7397) (156.0198, 193.7606) (155.8861, 193.7767) (155.7857, 193.7885) (155.7187, 193.7962) (155.6851, 193.8) knots 0 0 0 0 0 0 0.01428571 0.02857143 0.04285714 0.05714286 0.07142857 0.08571429 0.1 0.11428571 0.12857143 0.14285714 0.15714286 0.17142857 0.18571429 0.2 0.21428571 0.22857143 0.24285714 0.25714286 0.27142857 0.28571429 0.3 0.31428571 0.32857143 0.34285714 0.35714286 0.37142857 0.38571429 0.4 0.41428571 0.42857143 0.44285714 0.45714286 0.47142857 0.48571429 0.5 0.51428571 0.52857143 0.54285714 0.55714286 0.57142857 0.58571429 0.6 0.61428571 0.62857143 0.64285714 0.65714286 0.67142857 0.68571429 0.7 0.71428571 0.72857143 0.74285714 0.75714286 0.77142857 0.78571429 0.8 0.81428571 0.82857143 0.84285714 0.85714286 0.87142857 0.88571429 0.9 0.91428571 0.92857143 0.94285714 0.95714286 0.97142857 0.98571429 1 1 1 1 1 1
  line L10723 (166.3167, 190.3263) -> (166.2935, 190.3467) construction
  line L10724 (166.2935, 190.3467) -> (166.2466, 190.3868) construction
  line L10725 (166.2466, 190.3868) -> (166.1747, 190.4451) construction
  line L10726 (166.1747, 190.4451) -> (166.076, 190.5192) construction
  line L10727 (166.076, 190.5192) -> (165.9487, 190.6066) construction
  line L10728 (165.9487, 190.6066) -> (165.8185, 190.6904) construction
  line L10729 (165.8185, 190.6904) -> (165.6866, 190.772) construction
  line L10730 (165.6866, 190.772) -> (165.5538, 190.8524) construction
  line L10731 (165.5538, 190.8524) -> (165.4203, 190.932) construction
  line L10732 (165.4203, 190.932) -> (165.2862, 191.0107) construction
  line L10733 (165.2862, 191.0107) -> (165.1513, 191.0883) construction
  line L10734 (165.1513, 191.0883) -> (165.0152, 191.1642) construction
  line L10735 (165.0152, 191.1642) -> (164.8777, 191.2383) construction
  line L10736 (164.8777, 191.2383) -> (164.739, 191.3106) construction
  line L10737 (164.739, 191.3106) -> (164.5991, 191.3813) construction
  line L10738 (164.5991, 191.3813) -> (164.4582, 191.4504) construction
  line L10739 (164.4582, 191.4504) -> (164.3164, 191.5184) construction
  line L10740 (164.3164, 191.5184) -> (164.1739, 191.5853) construction
  line L10741 (164.1739, 191.5853) -> (164.0308, 191.6512) construction
  line L10742 (164.0308, 191.6512) -> (163.887, 191.716) construction
  line L10743 (163.887, 191.716) -> (163.7425, 191.7798) construction
  line L10744 (163.7425, 191.7798) -> (163.5973, 191.8424) construction
  line L10745 (163.5973, 191.8424) -> (163.4513, 191.9039) construction
  line L10746 (163.4513, 191.9039) -> (163.3046, 191.9642) construction
  line L10747 (163.3046, 191.9642) -> (163.1571, 192.0234) construction
  line L10748 (163.1571, 192.0234) -> (163.009, 192.0815) construction
  line L10749 (163.009, 192.0815) -> (162.8603, 192.1386) construction
  line L10750 (162.8603, 192.1386) -> (162.711, 192.1947) construction
  line L10751 (162.711, 192.1947) -> (162.5611, 192.2499) construction
  line L10752 (162.5611, 192.2499) -> (162.4106, 192.3041) construction
  line L10753 (162.4106, 192.3041) -> (162.2596, 192.3574) construction
  line L10754 (162.2596, 192.3574) -> (162.108, 192.4097) construction
  line L10755 (162.108, 192.4097) -> (161.9559, 192.461) construction
  line L10756 (161.9559, 192.461) -> (161.8032, 192.5114) construction
  line L10757 (161.8032, 192.5114) -> (161.65, 192.5608) construction
  line L10758 (161.65, 192.5608) -> (161.4962, 192.6094) construction
  line L10759 (161.4962, 192.6094) -> (161.342, 192.657) construction
  line L10760 (161.342, 192.657) -> (161.1873, 192.7037) construction
  line L10761 (161.1873, 192.7037) -> (161.0321, 192.7495) construction
  line L10762 (161.0321, 192.7495) -> (160.8764, 192.7945) construction
  line L10763 (160.8764, 192.7945) -> (160.7202, 192.8386) construction
  line L10764 (160.7202, 192.8386) -> (160.5636, 192.8818) construction
  line L10765 (160.5636, 192.8818) -> (160.4065, 192.9241) construction
  line L10766 (160.4065, 192.9241) -> (160.249, 192.9656) construction
  line L10767 (160.249, 192.9656) -> (160.0911, 193.0063) construction
  line L10768 (160.0911, 193.0063) -> (159.9327, 193.0461) construction
  line L10769 (159.9327, 193.0461) -> (159.7739, 193.085) construction
  line L10770 (159.7739, 193.085) -> (159.6147, 193.1231) construction
  line L10771 (159.6147, 193.1231) -> (159.4551, 193.1604) construction
  line L10772 (159.4551, 193.1604) -> (159.2951, 193.1969) construction
  line L10773 (159.2951, 193.1969) -> (159.1347, 193.2326) construction
  line L10774 (159.1347, 193.2326) -> (158.9739, 193.2674) construction
  line L10775 (158.9739, 193.2674) -> (158.8127, 193.3015) construction
  line L10776 (158.8127, 193.3015) -> (158.6511, 193.3347) construction
  line L10777 (158.6511, 193.3347) -> (158.4892, 193.3672) construction
  line L10778 (158.4892, 193.3672) -> (158.3269, 193.3988) construction
  line L10779 (158.3269, 193.3988) -> (158.1643, 193.4297) construction
  line L10780 (158.1643, 193.4297) -> (158.0013, 193.4597) construction
  line L10781 (158.0013, 193.4597) -> (157.838, 193.489) construction
  line L10782 (157.838, 193.489) -> (157.6743, 193.5175) construction
  line L10783 (157.6743, 193.5175) -> (157.5103, 193.5453) construction
  line L10784 (157.5103, 193.5453) -> (157.3459, 193.5723) construction
  line L10785 (157.3459, 193.5723) -> (157.1812, 193.5984) construction
  line L10786 (157.1812, 193.5984) -> (157.0162, 193.6239) construction
  line L10787 (157.0162, 193.6239) -> (156.8509, 193.6486) construction
  line L10788 (156.8509, 193.6486) -> (156.6853, 193.6725) construction
  line L10789 (156.6853, 193.6725) -> (156.5194, 193.6956) construction
  line L10790 (156.5194, 193.6956) -> (156.3531, 193.718) construction
  line L10791 (156.3531, 193.718) -> (156.1866, 193.7397) construction
  line L10792 (156.1866, 193.7397) -> (156.0198, 193.7606) construction
  line L10793 (156.0198, 193.7606) -> (155.8861, 193.7767) construction
  line L10794 (155.8861, 193.7767) -> (155.7857, 193.7885) construction
  line L10795 (155.7857, 193.7885) -> (155.7187, 193.7962) construction
  line L10796 (155.7187, 193.7962) -> (155.6851, 193.8) construction
  arc A283 (140.7205, 152.2563) -> (140.7205, 147.7437) centre (212.132, 150) ccw